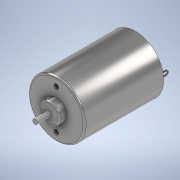
# Autodesk Inventor part: R370-25120
Saved by Autodesk Inventor 2020 (Build 240168000, 168)
## iProperties
Created: 2019-12-09
Part Number: R370-25120
Material: Stainless Steel, 440C
Document SubType Name: Modeling
Designer: salll
Density: 7.75 g/cm^3
Appearance: Semi-Polished
Author: salll
Autodesk Inventor part; units mm, degrees
ref_plane "YZ Plane" through (0, 0, 0) normal (1, 0, 0) x (0, 1, 0)
ref_plane "XZ Plane" through (0, 0, 0) normal (0, 1, 0) x (-1, 0, 0)
ref_plane "XY Plane" through (0, 0, 0) normal (0, 0, 1) x (1, 0, 0)
sketch "Эскиз1" plane through (0, 0, 0) normal (0, 0, 1) x (1, 0, 0)
  circle A0 centre (0, 0) radius 17.85
  dimension "d37" = 35.7
  constraints: 1 centre point, 1 coincident
  measures "d37" diameter of A0
extrude "Выдавливание1" add sketch "Эскиз1" along normal blind 50
sketch "Sketch7" plane through (0, 0, 50) normal (0, 0, 1) x (1, 0, 0)
  circle A0 centre (0, 0) radius 6.5
  dimension "d40" = 13
  constraints: 1 centre point, 1 coincident
  measures "d40" diameter of A0
extrude "Extrusion7" add sketch "Sketch7" along normal blind 4.5
sketch "Sketch8" plane through (0, 0, 54.5) normal (0, 0, 1) x (1, 0, 0)
  circle A0 centre (0, 0) radius 1.5
  dimension "d43" = 3
  constraints: 1 centre point, 1 coincident
  measures "d43" diameter of A0
extrude "Extrusion8" add sketch "Sketch8" along normal blind 9
sketch "Sketch10" plane through (0, 0, 50) normal (0, 0, 1) x (1, 0, 0)
  circle A0 centre (0, 12.5) radius 1.5
  circle A1 centre (0, -12.5) radius 1.5
  point P0 (0, 0)
  dimension "d53" = 3
  dimension "d54" = 3
  dimension "d58" = 12.5
  dimension "d59" = 12.5
  constraints: 2 centre point, 2 coincident
  measures "d53" diameter of A0
  measures "d54" diameter of A1
  measures "d58" distance of point (0, 0) point (0, -12.5)
  measures "d59" distance of point (0, 0) point (0, 12.5)
extrude "Extrusion9" cut sketch "Sketch10" against normal blind 5
thread "Thread1" size "M3x0.5" class "6H" standard "ANSI Metric M Profile" full length
thread "Thread2" size "M3x0.5" class "6H" standard "ANSI Metric M Profile" full length
sketch "Sketch12" plane through (0, 0, 0) normal (0, 0, -1) x (-1, 0, 0)
  circle A0 centre (0, 0) radius 6.5
  dimension "d67" = 13
  constraints: 1 centre point, 1 coincident
  measures "d67" diameter of A0
extrude "Extrusion10" add sketch "Sketch12" along normal blind 3
sketch "Sketch13" plane through (0, 0, -3) normal (0, 0, -1) x (-1, 0, 0)
  circle A0 centre (0, 0) radius 1.25
  dimension "d70" = 2.5
  constraints: 1 centre point, 1 coincident
  measures "d70" diameter of A0
extrude "Extrusion11" add sketch "Sketch13" along normal blind 0.5
fillet "Fillet3" radius 1 1 edges at (6.5, 0, -3)
fillet "Fillet4" radius 0.3 1 edges at (1.25, 0, -3.5)
fillet "Fillet5" radius 1 1 edges at (-6.5, 0, 54.5)
sketch "Sketch14" plane through (0, 0, 0) normal (0, 0, -1) x (-1, 0, 0)
  line L0 (14.85, -1.5) -> (14.35, -1.5)
  line L1 (14.35, -1.5) -> (14.35, 1.5)
  line L2 (14.35, 1.5) -> (14.85, 1.5)
  line L3 (14.85, 1.5) -> (14.85, -1.5)
  line L4 (-14.35, -1.5) -> (-14.85, -1.5)
  line L5 (-14.85, -1.5) -> (-14.85, 1.5)
  line L6 (-14.85, 1.5) -> (-14.35, 1.5)
  line L7 (-14.35, 1.5) -> (-14.35, -1.5)
  line L8 (0, 0) -> (18.9187, 0)
  circle A0 centre (0, 0) radius 1.5 projected
  line L9 (0, 0) -> (-19.0249, 0)
  dimension "d76" = 0.5
  dimension "d77" = 0.5
  dimension "d78" = 28.7
  dimension "d79" = 14.35
  dimension "d80" = 3
  constraints: 20 end point, 4 horizontal, 4 parallel, 2 perpendicular, 1 point on line, 2 other
  measures "d76" distance of L1.end L2.end
  measures "d77" distance of L5.end L6.end
  measures "d78" distance between parallel lines of L7 L1
  measures "d79" distance from line of L8.start L1
  measures "d80" distance of L0.end L1.end
extrude "Extrusion12" add sketch "Sketch14" along normal blind 6 contours L0 L1 L8 L3 | L8 L1 L2 L3 | L4 L5 L9 L7 | L9 L5 L6 L7
fillet "Fillet6" radius 1.5 4 edges at (-14.6, -1.5, -6) (-14.6, 1.5, -6) (14.6, -1.5, -6) (14.6, 1.5, -6)
sketch "Sketch15" plane through (-14.85, -1.5, 0) normal (-1, 0, 0) x (0, 0, 1)
  line L0 (-1, 0.5) -> (-4.5, 0.5)
  line L1 (-4.5, 2.5) -> (-1, 2.5)
  line L2 (-1, 2.5) -> (-1, 0.5)
  line L3 (0, 0) -> (-4.5, 0) projected
  line L4 (0, 3) -> (-4.5, 3) projected
  line L5 (0, -16.35) -> (0, 19.35) projected
  arc A0 (-4.5, 2.5) -> (-4.5, 0.5) centre (-4.5, 1.5) ccw
  point P0 (0, 1.5)
  dimension "d84" = 0.5
  dimension "d85" = 0.5
  dimension "d86" = 1
  dimension "d87" = 3.5
  dimension "d88" = 3.5
  dimension "d89" = 1
  constraints: 6 end point, 2 point on circle, 1 centre point, 1 horizontal, 1 parallel
  measures "d84" distance between parallel lines of L0 L3
  measures "d85" distance between parallel lines of L1 L4
  measures "d86" distance between parallel lines of L5 L2
  measures "d87" distance of L0.start L0.end
  measures "d88" distance of L1.start L1.end
  measures "d89" radius of A0
extrude "Extrusion13" cut sketch "Sketch15" against normal blind 1
sketch "Sketch16" plane through (14.85, -1.5, 0) normal (1, 0, 0) x (0, 0, -1)
  line L0 (1, 2.5) -> (1, 0.5) projected
  line L1 (1, 2.5) -> (4.5, 2.5) projected
  line L2 (1, 0.5) -> (4.5, 0.5)
  line L3 (4.5, 2.5) -> (1, 2.5)
  line L4 (1, 2.5) -> (1, 0.5)
  arc A0 (4.5, 0.5) -> (4.5, 2.5) centre (4.5, 1.5) ccw projected
  arc A1 (4.5, 0.5) -> (4.5, 2.5) centre (4.5, 1.5) ccw
  point P0 (0, 1.5)
  dimension "d92" = 1
  constraints: 6 end point, 2 point on circle, 1 centre point, 1 horizontal, 1 parallel
  measures "d92" radius of A1
extrude "Extrusion14" cut sketch "Sketch16" against normal blind 1
fillet "Fillet7" radius 1 1 edges at (-17.85, 0, 50)
